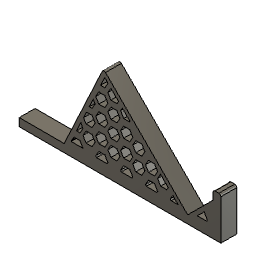
textbook holder fusion (Autodesk Fusion 360 design; units mm, degrees)
Autodesk Fusion 360 part; units mm, degrees
ref_plane "WorkPlane1" through (0, 0, 12.125) normal (0.707107, 0.707107, 0) x (0, 0, 1)
sketch "Sketch3" plane through (0, 0, 0) normal (0.707107, 0.707107, 0) x (0, 0, 1)
  line L0 (-200, 150) -> (200, 150)
  line L1 (200, 150) -> (200, -150)
  line L2 (200, -150) -> (-200, -150)
  line L3 (-200, -150) -> (-200, 150)
  line L4 (-200, 150) -> (200, -150) construction
  line L5 (200, 150) -> (-200, -150) construction
  point P0 (0, 116.066)
  point P1 (0, 116.066)
  dimension "d2" = 400
  dimension "d3" = 300
  constraint horizontal L0
  constraint perpendicular L0 L1
  constraint parallel L0 L2
  constraint parallel L1 L3
  constraint coincident L4 origin
  constraint coincident L5 origin
  measures "d2" distance of L1.end L2.end
  measures "d3" distance of L0.end L1.end
extrude "Extrude1" add sketch "Sketch3" along normal blind 45 makes body 1
sketch "Sketch4" plane through (0, 0, 0) normal (0, 1, 0) x (1, 0, 0)
  line L0 (106.066, 200) -> (106.066, -200)
move_body "Move1" bodies 1 to x (1, 0, 0) y (0, 1, 0) z (0, 0, 1) at (0, 106.066, 0)
move_body "Move2" bodies 1 to x (1, 0, 0) y (0, 1, 0) z (0, 0, 1) at (0, 10, 0)
sketch "Sketch5" plane through (0, 0, 0) normal (0, 1, 0) x (1, 0, 0)
  line L0 (106.066, -200) -> (-106.066, -200)
  line L1 (-106.066, 200) -> (106.066, 200)
  line L2 (106.066, -200) -> (137.8858, -200)
  line L3 (106.066, 200) -> (137.8858, 200)
  line L4 (-106.066, -200) -> (-106.066, 200)
  line L5 (137.8858, -200) -> (137.8858, 200)
  line L6 (-106.066, -180) -> (147.8858, -180)
  line L7 (147.8858, 180) -> (-106.066, 180)
  line L8 (137.8858, 200) -> (147.8858, 200)
  line L9 (137.8858, -200) -> (147.8858, -200)
  line L10 (147.8858, -200) -> (147.8858, 200)
  dimension "d9" = 20
  dimension "d10" = 20
  dimension "d13" = 10
  dimension "d14" = 10
  constraint coincident L4 L6.start
  constraint perpendicular L5 L6
  constraint coincident L4 L7.end
  constraint perpendicular L4 L7
  constraint coincident L3.end L5.end
  constraint perpendicular L5 L8
  constraint coincident L2.end L5.start
  constraint perpendicular L5 L9
  constraint coincident L10 L6.end
  constraint coincident L10 L7.start
  measures "d9" distance of L1 L7
  measures "d10" distance of L0 L6
  measures "d13" distance of L3.end L8.end
  measures "d14" distance of L2.end L9.end
extrude "Extrude2" add sketch "Sketch5" along normal blind 10 separate body contours L1 L3 L4 L5 L7 | L5 L7 L8 L10 makes body 2
sketch "Sketch6" plane through (0, 10, 0) normal (0, 1, 0) x (-1, 0, 0)
  line L0 (-147.8858, -180) -> (-147.8858, -200)
  line L1 (-147.8858, -200) -> (106.066, -200)
  line L2 (106.066, -200) -> (106.066, -180)
  line L3 (106.066, -180) -> (-147.8858, -180)
  line L4 (-147.8858, -180) -> (-137.8858, -180)
  line L5 (-137.8858, -180) -> (-137.8858, -200)
  line L6 (-137.8858, -200) -> (-147.8858, -200)
  line L7 (-147.8858, -200) -> (-147.8858, -180)
  dimension "d15" = 10
  constraint horizontal L4
  constraint vertical L5
  constraint horizontal L6
  constraint vertical L7
  constraint coincident L0.start L3.end
  measures "d15" distance of L0.start L4.end
extrude "Extrude3" add sketch "Sketch6" along normal blind 43.18 contours L0 L1 L3 L4 L5 L6 L7 bodies 2
sketch "Sketch7" plane through (0, 10, 0) normal (0, 1, 0) x (-1, 0, 0)
  line L0 (-137.8858, -180) -> (-137.8858, -200)
  line L1 (-137.8858, -200) -> (106.066, -200)
  line L2 (106.066, -180) -> (-137.8858, -180)
  line L3 (106.066, -180) -> (-137.8858, -180)
  line L4 (-137.8858, -200) -> (106.066, -200)
  line L5 (-133.1972, -180) -> (-133.1972, -200)
  line L6 (-123.4094, -200) -> (-123.4094, -180)
  line L7 (-123.4094, -184.92) -> (-133.1972, -184.92)
  line L8 (-133.1972, -190) -> (-123.4094, -190)
  line L9 (-123.4094, -195.08) -> (-133.1972, -195.08)
  line L10 (-133.1972, -180) -> (-123.4094, -180)
  line L11 (-128.3033, -180) -> (-128.3033, -200)
  line L12 (106.066, -200) -> (106.066, -180)
  point P0 (-128.3033, -184.92)
  point P1 (-128.3033, -190)
  point P2 (-128.3033, -195.08)
  dimension "d18" = 5.08
  dimension "d19" = 5.08
  constraint coincident L2.start L3.start
  constraint coincident L0.start L2.end
  constraint coincident L0.end L1.start
  constraint coincident L1.end L4.end
  constraint coincident L2 L5.start
  constraint coincident L4 L5.end
  constraint perpendicular L4 L5
  constraint coincident L1 L6.start
  constraint coincident L2 L6.end
  constraint perpendicular L2 L6
  constraint coincident L6 L7.start
  constraint coincident L5 L7.end
  constraint perpendicular L5 L7
  constraint midpoint L5 L8.start
  constraint midpoint L6 L8.end
  constraint coincident L6 L9.start
  constraint coincident L5 L9.end
  constraint perpendicular L5 L9
  constraint midpoint L10 L11.start
  constraint coincident L1 L11.end
  constraint perpendicular L1 L11
  constraint midpoint L7 P0
  constraint midpoint L8 P1
  constraint midpoint L9 P2
  measures "d18" distance of L7 L8
  measures "d19" distance of L8 L9
ref_plane "WorkPlane2" through (128.3033, 10, -190) normal (0, 0, -1) x (-1, 0, 0)
sketch "Sketch8" plane through (128.3033, 10, -190) normal (0, 0, -1) x (-1, 0, 0)
  line L0 (22.2373, 0) -> (-9.5825, 31.8198)
  line L1 (-9.5825, 0) -> (-9.5825, 43.18)
  line L2 (-9.5825, 0) -> (234.3693, 0)
  line L3 (234.3693, 212.132) -> (22.2373, 0)
  line L4 (-9.5825, 0) -> (234.3693, 0)
  line L5 (128.3033, 106.066) -> (22.2373, 0)
  line L6 (128.3033, 106.066) -> (177.7627, 0)
  dimension "d24" = 45
  dimension "d25" = 150
  dimension "d26" = 65
  constraint coincident L4 L0.start
  constraint coincident L0.start L3.end
  constraint coincident L2 L6.end
  measures "d24" angle of L4 L5
  measures "d25" distance of L5.start L0.start
  measures "d26" angle of L4 L6
extrude "Extrude5" add sketch "Sketch8" along normal mid plane 20 bodies 2
sketch "Sketch9" plane through (0, 0, -200) normal (0, 0, -1) x (-1, 0, 0)
  line L0 (49.4594, 10) -> (0, 116.066)
  line L1 (0, 116.066) -> (-106.066, 10)
  line L2 (53.2694, 3.4009) -> (57.0794, 10)
  line L3 (57.0794, 10) -> (53.2694, 16.5991)
  line L4 (53.2694, 16.5991) -> (45.6494, 16.5991)
  line L5 (45.6494, 16.5991) -> (41.8394, 10)
  line L6 (41.8394, 10) -> (45.6494, 3.4009)
  line L7 (45.6494, 3.4009) -> (53.2694, 3.4009)
  line L8 (41.611, 15) -> (-1.5137, 107.4812)
  line L9 (-1.5137, 107.4812) -> (-93.9949, 15)
  line L10 (-93.9949, 15) -> (41.611, 15)
  line L11 (-106.066, 10) -> (-137.8858, 41.8198)
  line L12 (-132.8858, 15) -> (-118.1371, 15)
  line L13 (-118.1371, 15) -> (-132.8858, 29.7487)
  line L14 (-132.8858, 29.7487) -> (-132.8858, 15)
  line L15 (29.6006, 10) -> (37.2206, 10)
  line L16 (37.2206, 10) -> (41.0306, 16.5991)
  line L17 (41.0306, 16.5991) -> (37.2206, 23.1982)
  line L18 (37.2206, 23.1982) -> (29.6006, 23.1982)
  line L19 (29.6006, 23.1982) -> (25.7906, 16.5991)
  line L20 (25.7906, 16.5991) -> (29.6006, 10)
  line L21 (106.066, 0) -> (-147.8858, 0)
  line L22 (45.6494, 16.5991) -> (23.7329, 16.5991)
  line L23 (14.3227, 16.5991) -> (10.5127, 10)
  line L24 (10.5127, 10) -> (14.3227, 3.4009)
  line L25 (14.3227, 3.4009) -> (21.9427, 3.4009)
  line L26 (21.9427, 3.4009) -> (25.7527, 10)
  line L27 (25.7527, 10) -> (21.9427, 16.5991)
  line L28 (21.9427, 16.5991) -> (14.3227, 16.5991)
  line L29 (-17.0039, 16.5991) -> (-20.8139, 10)
  line L30 (-20.8139, 10) -> (-17.0039, 3.4009)
  line L31 (-17.0039, 3.4009) -> (-9.3839, 3.4009)
  line L32 (-9.3839, 3.4009) -> (-5.5739, 10)
  line L33 (-5.5739, 10) -> (-9.3839, 16.5991)
  line L34 (-9.3839, 16.5991) -> (-17.0039, 16.5991)
  line L35 (-48.3306, 16.5991) -> (-52.1406, 10)
  line L36 (-52.1406, 10) -> (-48.3306, 3.4009)
  line L37 (-48.3306, 3.4009) -> (-40.7106, 3.4009)
  line L38 (-40.7106, 3.4009) -> (-36.9006, 10)
  line L39 (-36.9006, 10) -> (-40.7106, 16.5991)
  line L40 (-40.7106, 16.5991) -> (-48.3306, 16.5991)
  line L41 (-79.6573, 16.5991) -> (-83.4673, 10)
  line L42 (-83.4673, 10) -> (-79.6573, 3.4009)
  line L43 (-79.6573, 3.4009) -> (-72.0373, 3.4009)
  line L44 (-72.0373, 3.4009) -> (-68.2273, 10)
  line L45 (-68.2273, 10) -> (-72.0373, 16.5991)
  line L46 (-72.0373, 16.5991) -> (-79.6573, 16.5991)
  line L47 (-110.9839, 16.5991) -> (-114.7939, 10)
  line L48 (-114.7939, 10) -> (-110.9839, 3.4009)
  line L49 (-110.9839, 3.4009) -> (-103.3639, 3.4009)
  line L50 (-103.3639, 3.4009) -> (-99.5539, 10)
  line L51 (-99.5539, 10) -> (-103.3639, 16.5991)
  line L52 (-103.3639, 16.5991) -> (-110.9839, 16.5991)
  line L53 (-142.3106, 16.5991) -> (-146.1206, 10)
  line L54 (-146.1206, 10) -> (-142.3106, 3.4009)
  line L55 (-142.3106, 3.4009) -> (-134.6906, 3.4009)
  line L56 (-134.6906, 3.4009) -> (-130.8806, 10)
  line L57 (-130.8806, 10) -> (-134.6906, 16.5991)
  line L58 (-134.6906, 16.5991) -> (-142.3106, 16.5991)
  line L59 (45.6494, 37.4271) -> (41.8394, 30.828)
  line L60 (41.8394, 30.828) -> (45.6494, 24.2289)
  line L61 (45.6494, 24.2289) -> (53.2694, 24.2289)
  line L62 (53.2694, 24.2289) -> (57.0794, 30.828)
  line L63 (57.0794, 30.828) -> (53.2694, 37.4271)
  line L64 (53.2694, 37.4271) -> (45.6494, 37.4271)
  line L65 (14.3227, 37.4271) -> (10.5127, 30.828)
  line L66 (10.5127, 30.828) -> (14.3227, 24.2289)
  line L67 (14.3227, 24.2289) -> (21.9427, 24.2289)
  line L68 (21.9427, 24.2289) -> (25.7527, 30.828)
  line L69 (25.7527, 30.828) -> (21.9427, 37.4271)
  line L70 (21.9427, 37.4271) -> (14.3227, 37.4271)
  line L71 (-17.0039, 37.4271) -> (-20.8139, 30.828)
  line L72 (-20.8139, 30.828) -> (-17.0039, 24.2289)
  line L73 (-17.0039, 24.2289) -> (-9.3839, 24.2289)
  line L74 (-9.3839, 24.2289) -> (-5.5739, 30.828)
  line L75 (-5.5739, 30.828) -> (-9.3839, 37.4271)
  line L76 (-9.3839, 37.4271) -> (-17.0039, 37.4271)
  line L77 (-48.3306, 37.4271) -> (-52.1406, 30.828)
  line L78 (-52.1406, 30.828) -> (-48.3306, 24.2289)
  line L79 (-48.3306, 24.2289) -> (-40.7106, 24.2289)
  line L80 (-40.7106, 24.2289) -> (-36.9006, 30.828)
  line L81 (-36.9006, 30.828) -> (-40.7106, 37.4271)
  line L82 (-40.7106, 37.4271) -> (-48.3306, 37.4271)
  line L83 (-79.6573, 37.4271) -> (-83.4673, 30.828)
  line L84 (-83.4673, 30.828) -> (-79.6573, 24.2289)
  line L85 (-79.6573, 24.2289) -> (-72.0373, 24.2289)
  line L86 (-72.0373, 24.2289) -> (-68.2273, 30.828)
  line L87 (-68.2273, 30.828) -> (-72.0373, 37.4271)
  line L88 (-72.0373, 37.4271) -> (-79.6573, 37.4271)
  line L89 (-110.9839, 37.4271) -> (-114.7939, 30.828)
  line L90 (-114.7939, 30.828) -> (-110.9839, 24.2289)
  line L91 (-110.9839, 24.2289) -> (-103.3639, 24.2289)
  line L92 (-103.3639, 24.2289) -> (-99.5539, 30.828)
  line L93 (-99.5539, 30.828) -> (-103.3639, 37.4271)
  line L94 (-103.3639, 37.4271) -> (-110.9839, 37.4271)
  line L95 (-142.3106, 37.4271) -> (-146.1206, 30.828)
  line L96 (-146.1206, 30.828) -> (-142.3106, 24.2289)
  line L97 (-142.3106, 24.2289) -> (-134.6906, 24.2289)
  line L98 (-134.6906, 24.2289) -> (-130.8806, 30.828)
  line L99 (-130.8806, 30.828) -> (-134.6906, 37.4271)
  line L100 (-134.6906, 37.4271) -> (-142.3106, 37.4271)
  line L101 (45.6494, 58.2551) -> (41.8394, 51.656)
  line L102 (41.8394, 51.656) -> (45.6494, 45.0569)
  line L103 (45.6494, 45.0569) -> (53.2694, 45.0569)
  line L104 (53.2694, 45.0569) -> (57.0794, 51.656)
  line L105 (57.0794, 51.656) -> (53.2694, 58.2551)
  line L106 (53.2694, 58.2551) -> (45.6494, 58.2551)
  line L107 (14.3227, 58.2551) -> (10.5127, 51.656)
  line L108 (10.5127, 51.656) -> (14.3227, 45.0569)
  line L109 (14.3227, 45.0569) -> (21.9427, 45.0569)
  line L110 (21.9427, 45.0569) -> (25.7527, 51.656)
  line L111 (25.7527, 51.656) -> (21.9427, 58.2551)
  line L112 (21.9427, 58.2551) -> (14.3227, 58.2551)
  line L113 (-17.0039, 58.2551) -> (-20.8139, 51.656)
  line L114 (-20.8139, 51.656) -> (-17.0039, 45.0569)
  line L115 (-17.0039, 45.0569) -> (-9.3839, 45.0569)
  line L116 (-9.3839, 45.0569) -> (-5.5739, 51.656)
  line L117 (-5.5739, 51.656) -> (-9.3839, 58.2551)
  line L118 (-9.3839, 58.2551) -> (-17.0039, 58.2551)
  line L119 (-48.3306, 58.2551) -> (-52.1406, 51.656)
  line L120 (-52.1406, 51.656) -> (-48.3306, 45.0569)
  line L121 (-48.3306, 45.0569) -> (-40.7106, 45.0569)
  line L122 (-40.7106, 45.0569) -> (-36.9006, 51.656)
  line L123 (-36.9006, 51.656) -> (-40.7106, 58.2551)
  line L124 (-40.7106, 58.2551) -> (-48.3306, 58.2551)
  line L125 (-79.6573, 58.2551) -> (-83.4673, 51.656)
  line L126 (-83.4673, 51.656) -> (-79.6573, 45.0569)
  line L127 (-79.6573, 45.0569) -> (-72.0373, 45.0569)
  line L128 (-72.0373, 45.0569) -> (-68.2273, 51.656)
  line L129 (-68.2273, 51.656) -> (-72.0373, 58.2551)
  line L130 (-72.0373, 58.2551) -> (-79.6573, 58.2551)
  line L131 (-110.9839, 58.2551) -> (-114.7939, 51.656)
  line L132 (-114.7939, 51.656) -> (-110.9839, 45.0569)
  line L133 (-110.9839, 45.0569) -> (-103.3639, 45.0569)
  line L134 (-103.3639, 45.0569) -> (-99.5539, 51.656)
  line L135 (-99.5539, 51.656) -> (-103.3639, 58.2551)
  line L136 (-103.3639, 58.2551) -> (-110.9839, 58.2551)
  line L137 (-142.3106, 58.2551) -> (-146.1206, 51.656)
  line L138 (-146.1206, 51.656) -> (-142.3106, 45.0569)
  line L139 (-142.3106, 45.0569) -> (-134.6906, 45.0569)
  line L140 (-134.6906, 45.0569) -> (-130.8806, 51.656)
  line L141 (-130.8806, 51.656) -> (-134.6906, 58.2551)
  line L142 (-134.6906, 58.2551) -> (-142.3106, 58.2551)
  line L143 (45.6494, 79.0831) -> (41.8394, 72.484)
  line L144 (41.8394, 72.484) -> (45.6494, 65.8849)
  line L145 (45.6494, 65.8849) -> (53.2694, 65.8849)
  line L146 (53.2694, 65.8849) -> (57.0794, 72.484)
  line L147 (57.0794, 72.484) -> (53.2694, 79.0831)
  line L148 (53.2694, 79.0831) -> (45.6494, 79.0831)
  line L149 (14.3227, 79.0831) -> (10.5127, 72.484)
  line L150 (10.5127, 72.484) -> (14.3227, 65.8849)
  line L151 (14.3227, 65.8849) -> (21.9427, 65.8849)
  line L152 (21.9427, 65.8849) -> (25.7527, 72.484)
  line L153 (25.7527, 72.484) -> (21.9427, 79.0831)
  line L154 (21.9427, 79.0831) -> (14.3227, 79.0831)
  line L155 (-17.0039, 79.0831) -> (-20.8139, 72.484)
  line L156 (-20.8139, 72.484) -> (-17.0039, 65.8849)
  line L157 (-17.0039, 65.8849) -> (-9.3839, 65.8849)
  line L158 (-9.3839, 65.8849) -> (-5.5739, 72.484)
  line L159 (-5.5739, 72.484) -> (-9.3839, 79.0831)
  line L160 (-9.3839, 79.0831) -> (-17.0039, 79.0831)
  line L161 (-48.3306, 79.0831) -> (-52.1406, 72.484)
  line L162 (-52.1406, 72.484) -> (-48.3306, 65.8849)
  line L163 (-48.3306, 65.8849) -> (-40.7106, 65.8849)
  line L164 (-40.7106, 65.8849) -> (-36.9006, 72.484)
  line L165 (-36.9006, 72.484) -> (-40.7106, 79.0831)
  line L166 (-40.7106, 79.0831) -> (-48.3306, 79.0831)
  line L167 (-79.6573, 79.0831) -> (-83.4673, 72.484)
  line L168 (-83.4673, 72.484) -> (-79.6573, 65.8849)
  line L169 (-79.6573, 65.8849) -> (-72.0373, 65.8849)
  line L170 (-72.0373, 65.8849) -> (-68.2273, 72.484)
  line L171 (-68.2273, 72.484) -> (-72.0373, 79.0831)
  line L172 (-72.0373, 79.0831) -> (-79.6573, 79.0831)
  line L173 (-110.9839, 79.0831) -> (-114.7939, 72.484)
  line L174 (-114.7939, 72.484) -> (-110.9839, 65.8849)
  line L175 (-110.9839, 65.8849) -> (-103.3639, 65.8849)
  line L176 (-103.3639, 65.8849) -> (-99.5539, 72.484)
  line L177 (-99.5539, 72.484) -> (-103.3639, 79.0831)
  line L178 (-103.3639, 79.0831) -> (-110.9839, 79.0831)
  line L179 (-142.3106, 79.0831) -> (-146.1206, 72.484)
  line L180 (-146.1206, 72.484) -> (-142.3106, 65.8849)
  line L181 (-142.3106, 65.8849) -> (-134.6906, 65.8849)
  line L182 (-134.6906, 65.8849) -> (-130.8806, 72.484)
  line L183 (-130.8806, 72.484) -> (-134.6906, 79.0831)
  line L184 (-134.6906, 79.0831) -> (-142.3106, 79.0831)
  line L185 (45.6494, 99.9111) -> (41.8394, 93.312)
  line L186 (41.8394, 93.312) -> (45.6494, 86.7129)
  line L187 (45.6494, 86.7129) -> (53.2694, 86.7129)
  line L188 (53.2694, 86.7129) -> (57.0794, 93.312)
  line L189 (57.0794, 93.312) -> (53.2694, 99.9111)
  line L190 (53.2694, 99.9111) -> (45.6494, 99.9111)
  line L191 (14.3227, 99.9111) -> (10.5127, 93.312)
  line L192 (10.5127, 93.312) -> (14.3227, 86.7129)
  line L193 (14.3227, 86.7129) -> (21.9427, 86.7129)
  line L194 (21.9427, 86.7129) -> (25.7527, 93.312)
  line L195 (25.7527, 93.312) -> (21.9427, 99.9111)
  line L196 (21.9427, 99.9111) -> (14.3227, 99.9111)
  line L197 (-17.0039, 99.9111) -> (-20.8139, 93.312)
  line L198 (-20.8139, 93.312) -> (-17.0039, 86.7129)
  line L199 (-17.0039, 86.7129) -> (-9.3839, 86.7129)
  line L200 (-9.3839, 86.7129) -> (-5.5739, 93.312)
  line L201 (-5.5739, 93.312) -> (-9.3839, 99.9111)
  line L202 (-9.3839, 99.9111) -> (-17.0039, 99.9111)
  line L203 (-48.3306, 99.9111) -> (-52.1406, 93.312)
  line L204 (-52.1406, 93.312) -> (-48.3306, 86.7129)
  line L205 (-48.3306, 86.7129) -> (-40.7106, 86.7129)
  line L206 (-40.7106, 86.7129) -> (-36.9006, 93.312)
  line L207 (-36.9006, 93.312) -> (-40.7106, 99.9111)
  line L208 (-40.7106, 99.9111) -> (-48.3306, 99.9111)
  line L209 (-79.6573, 99.9111) -> (-83.4673, 93.312)
  line L210 (-83.4673, 93.312) -> (-79.6573, 86.7129)
  line L211 (-79.6573, 86.7129) -> (-72.0373, 86.7129)
  line L212 (-72.0373, 86.7129) -> (-68.2273, 93.312)
  line L213 (-68.2273, 93.312) -> (-72.0373, 99.9111)
  line L214 (-72.0373, 99.9111) -> (-79.6573, 99.9111)
  line L215 (-110.9839, 99.9111) -> (-114.7939, 93.312)
  line L216 (-114.7939, 93.312) -> (-110.9839, 86.7129)
  line L217 (-110.9839, 86.7129) -> (-103.3639, 86.7129)
  line L218 (-103.3639, 86.7129) -> (-99.5539, 93.312)
  line L219 (-99.5539, 93.312) -> (-103.3639, 99.9111)
  line L220 (-103.3639, 99.9111) -> (-110.9839, 99.9111)
  line L221 (-142.3106, 99.9111) -> (-146.1206, 93.312)
  line L222 (-146.1206, 93.312) -> (-142.3106, 86.7129)
  line L223 (-142.3106, 86.7129) -> (-134.6906, 86.7129)
  line L224 (-134.6906, 86.7129) -> (-130.8806, 93.312)
  line L225 (-130.8806, 93.312) -> (-134.6906, 99.9111)
  line L226 (-134.6906, 99.9111) -> (-142.3106, 99.9111)
  line L227 (45.6494, 120.7391) -> (41.8394, 114.14)
  line L228 (41.8394, 114.14) -> (45.6494, 107.5409)
  line L229 (45.6494, 107.5409) -> (53.2694, 107.5409)
  line L230 (53.2694, 107.5409) -> (57.0794, 114.14)
  line L231 (57.0794, 114.14) -> (53.2694, 120.7391)
  line L232 (53.2694, 120.7391) -> (45.6494, 120.7391)
  line L233 (14.3227, 120.7391) -> (10.5127, 114.14)
  line L234 (10.5127, 114.14) -> (14.3227, 107.5409)
  line L235 (14.3227, 107.5409) -> (21.9427, 107.5409)
  line L236 (21.9427, 107.5409) -> (25.7527, 114.14)
  line L237 (25.7527, 114.14) -> (21.9427, 120.7391)
  line L238 (21.9427, 120.7391) -> (14.3227, 120.7391)
  line L239 (-17.0039, 120.7391) -> (-20.8139, 114.14)
  line L240 (-20.8139, 114.14) -> (-17.0039, 107.5409)
  line L241 (-17.0039, 107.5409) -> (-9.3839, 107.5409)
  line L242 (-9.3839, 107.5409) -> (-5.5739, 114.14)
  line L243 (-5.5739, 114.14) -> (-9.3839, 120.7391)
  line L244 (-9.3839, 120.7391) -> (-17.0039, 120.7391)
  line L245 (-48.3306, 120.7391) -> (-52.1406, 114.14)
  line L246 (-52.1406, 114.14) -> (-48.3306, 107.5409)
  line L247 (-48.3306, 107.5409) -> (-40.7106, 107.5409)
  line L248 (-40.7106, 107.5409) -> (-36.9006, 114.14)
  line L249 (-36.9006, 114.14) -> (-40.7106, 120.7391)
  line L250 (-40.7106, 120.7391) -> (-48.3306, 120.7391)
  line L251 (-79.6573, 120.7391) -> (-83.4673, 114.14)
  line L252 (-83.4673, 114.14) -> (-79.6573, 107.5409)
  line L253 (-79.6573, 107.5409) -> (-72.0373, 107.5409)
  line L254 (-72.0373, 107.5409) -> (-68.2273, 114.14)
  line L255 (-68.2273, 114.14) -> (-72.0373, 120.7391)
  line L256 (-72.0373, 120.7391) -> (-79.6573, 120.7391)
  line L257 (-110.9839, 120.7391) -> (-114.7939, 114.14)
  line L258 (-114.7939, 114.14) -> (-110.9839, 107.5409)
  line L259 (-110.9839, 107.5409) -> (-103.3639, 107.5409)
  line L260 (-103.3639, 107.5409) -> (-99.5539, 114.14)
  line L261 (-99.5539, 114.14) -> (-103.3639, 120.7391)
  line L262 (-103.3639, 120.7391) -> (-110.9839, 120.7391)
  line L263 (-142.3106, 120.7391) -> (-146.1206, 114.14)
  line L264 (-146.1206, 114.14) -> (-142.3106, 107.5409)
  line L265 (-142.3106, 107.5409) -> (-134.6906, 107.5409)
  line L266 (-134.6906, 107.5409) -> (-130.8806, 114.14)
  line L267 (-130.8806, 114.14) -> (-134.6906, 120.7391)
  line L268 (-134.6906, 120.7391) -> (-142.3106, 120.7391)
  line L269 (-1.7261, 10) -> (5.8939, 10)
  line L270 (-5.5361, 16.5991) -> (-1.7261, 10)
  line L271 (5.8939, 23.1982) -> (-1.7261, 23.1982)
  line L272 (9.7039, 16.5991) -> (5.8939, 23.1982)
  line L273 (-1.7261, 23.1982) -> (-5.5361, 16.5991)
  line L274 (5.8939, 10) -> (9.7039, 16.5991)
  line L275 (-33.0527, 10) -> (-25.4327, 10)
  line L276 (-36.8627, 16.5991) -> (-33.0527, 10)
  line L277 (-25.4327, 23.1982) -> (-33.0527, 23.1982)
  line L278 (-21.6227, 16.5991) -> (-25.4327, 23.1982)
  line L279 (-33.0527, 23.1982) -> (-36.8627, 16.5991)
  line L280 (-25.4327, 10) -> (-21.6227, 16.5991)
  line L281 (-64.3794, 10) -> (-56.7594, 10)
  line L282 (-68.1894, 16.5991) -> (-64.3794, 10)
  line L283 (-56.7594, 23.1982) -> (-64.3794, 23.1982)
  line L284 (-52.9494, 16.5991) -> (-56.7594, 23.1982)
  line L285 (-64.3794, 23.1982) -> (-68.1894, 16.5991)
  line L286 (-56.7594, 10) -> (-52.9494, 16.5991)
  line L287 (-95.7061, 10) -> (-88.0861, 10)
  line L288 (-99.5161, 16.5991) -> (-95.7061, 10)
  line L289 (-88.0861, 23.1982) -> (-95.7061, 23.1982)
  line L290 (-84.2761, 16.5991) -> (-88.0861, 23.1982)
  line L291 (-95.7061, 23.1982) -> (-99.5161, 16.5991)
  line L292 (-88.0861, 10) -> (-84.2761, 16.5991)
  line L293 (-127.0327, 10) -> (-119.4127, 10)
  line L294 (-130.8427, 16.5991) -> (-127.0327, 10)
  line L295 (-119.4127, 23.1982) -> (-127.0327, 23.1982)
  line L296 (-115.6027, 16.5991) -> (-119.4127, 23.1982)
  line L297 (-127.0327, 23.1982) -> (-130.8427, 16.5991)
  line L298 (-119.4127, 10) -> (-115.6027, 16.5991)
  line L299 (-158.3594, 10) -> (-150.7394, 10)
  line L300 (-162.1694, 16.5991) -> (-158.3594, 10)
  line L301 (-150.7394, 23.1982) -> (-158.3594, 23.1982)
  line L302 (-146.9294, 16.5991) -> (-150.7394, 23.1982)
  line L303 (-158.3594, 23.1982) -> (-162.1694, 16.5991)
  line L304 (-150.7394, 10) -> (-146.9294, 16.5991)
  line L305 (29.6006, 31.59) -> (37.2206, 31.59)
  line L306 (25.7906, 38.1891) -> (29.6006, 31.59)
  line L307 (37.2206, 44.7882) -> (29.6006, 44.7882)
  line L308 (41.0306, 38.1891) -> (37.2206, 44.7882)
  line L309 (29.6006, 44.7882) -> (25.7906, 38.1891)
  line L310 (37.2206, 31.59) -> (41.0306, 38.1891)
  line L311 (-1.7261, 31.59) -> (5.8939, 31.59)
  line L312 (-5.5361, 38.1891) -> (-1.7261, 31.59)
  line L313 (5.8939, 44.7882) -> (-1.7261, 44.7882)
  line L314 (9.7039, 38.1891) -> (5.8939, 44.7882)
  line L315 (-1.7261, 44.7882) -> (-5.5361, 38.1891)
  line L316 (5.8939, 31.59) -> (9.7039, 38.1891)
  line L317 (-33.0527, 31.59) -> (-25.4327, 31.59)
  line L318 (-36.8627, 38.1891) -> (-33.0527, 31.59)
  line L319 (-25.4327, 44.7882) -> (-33.0527, 44.7882)
  line L320 (-21.6227, 38.1891) -> (-25.4327, 44.7882)
  line L321 (-33.0527, 44.7882) -> (-36.8627, 38.1891)
  line L322 (-25.4327, 31.59) -> (-21.6227, 38.1891)
  line L323 (-64.3794, 31.59) -> (-56.7594, 31.59)
  line L324 (-68.1894, 38.1891) -> (-64.3794, 31.59)
  line L325 (-56.7594, 44.7882) -> (-64.3794, 44.7882)
  line L326 (-52.9494, 38.1891) -> (-56.7594, 44.7882)
  line L327 (-64.3794, 44.7882) -> (-68.1894, 38.1891)
  line L328 (-56.7594, 31.59) -> (-52.9494, 38.1891)
  line L329 (-95.7061, 31.59) -> (-88.0861, 31.59)
  line L330 (-99.5161, 38.1891) -> (-95.7061, 31.59)
  line L331 (-88.0861, 44.7882) -> (-95.7061, 44.7882)
  line L332 (-84.2761, 38.1891) -> (-88.0861, 44.7882)
  line L333 (-95.7061, 44.7882) -> (-99.5161, 38.1891)
  line L334 (-88.0861, 31.59) -> (-84.2761, 38.1891)
  line L335 (-127.0327, 31.59) -> (-119.4127, 31.59)
  line L336 (-130.8427, 38.1891) -> (-127.0327, 31.59)
  line L337 (-119.4127, 44.7882) -> (-127.0327, 44.7882)
  line L338 (-115.6027, 38.1891) -> (-119.4127, 44.7882)
  line L339 (-127.0327, 44.7882) -> (-130.8427, 38.1891)
  line L340 (-119.4127, 31.59) -> (-115.6027, 38.1891)
  line L341 (-158.3594, 31.59) -> (-150.7394, 31.59)
  line L342 (-162.1694, 38.1891) -> (-158.3594, 31.59)
  line L343 (-150.7394, 44.7882) -> (-158.3594, 44.7882)
  line L344 (-146.9294, 38.1891) -> (-150.7394, 44.7882)
  line L345 (-158.3594, 44.7882) -> (-162.1694, 38.1891)
  line L346 (-150.7394, 31.59) -> (-146.9294, 38.1891)
  line L347 (29.6006, 53.18) -> (37.2206, 53.18)
  line L348 (25.7906, 59.7791) -> (29.6006, 53.18)
  line L349 (37.2206, 66.3782) -> (29.6006, 66.3782)
  line L350 (41.0306, 59.7791) -> (37.2206, 66.3782)
  line L351 (29.6006, 66.3782) -> (25.7906, 59.7791)
  line L352 (37.2206, 53.18) -> (41.0306, 59.7791)
  line L353 (-1.7261, 53.18) -> (5.8939, 53.18)
  line L354 (-5.5361, 59.7791) -> (-1.7261, 53.18)
  line L355 (5.8939, 66.3782) -> (-1.7261, 66.3782)
  line L356 (9.7039, 59.7791) -> (5.8939, 66.3782)
  line L357 (-1.7261, 66.3782) -> (-5.5361, 59.7791)
  line L358 (5.8939, 53.18) -> (9.7039, 59.7791)
  line L359 (-33.0527, 53.18) -> (-25.4327, 53.18)
  line L360 (-36.8627, 59.7791) -> (-33.0527, 53.18)
  line L361 (-25.4327, 66.3782) -> (-33.0527, 66.3782)
  line L362 (-21.6227, 59.7791) -> (-25.4327, 66.3782)
  line L363 (-33.0527, 66.3782) -> (-36.8627, 59.7791)
  line L364 (-25.4327, 53.18) -> (-21.6227, 59.7791)
  line L365 (-64.3794, 53.18) -> (-56.7594, 53.18)
  line L366 (-68.1894, 59.7791) -> (-64.3794, 53.18)
  line L367 (-56.7594, 66.3782) -> (-64.3794, 66.3782)
  line L368 (-52.9494, 59.7791) -> (-56.7594, 66.3782)
  line L369 (-64.3794, 66.3782) -> (-68.1894, 59.7791)
  line L370 (-56.7594, 53.18) -> (-52.9494, 59.7791)
  line L371 (-95.7061, 53.18) -> (-88.0861, 53.18)
  line L372 (-99.5161, 59.7791) -> (-95.7061, 53.18)
  line L373 (-88.0861, 66.3782) -> (-95.7061, 66.3782)
  line L374 (-84.2761, 59.7791) -> (-88.0861, 66.3782)
  line L375 (-95.7061, 66.3782) -> (-99.5161, 59.7791)
  line L376 (-88.0861, 53.18) -> (-84.2761, 59.7791)
  line L377 (-127.0327, 53.18) -> (-119.4127, 53.18)
  line L378 (-130.8427, 59.7791) -> (-127.0327, 53.18)
  line L379 (-119.4127, 66.3782) -> (-127.0327, 66.3782)
  line L380 (-115.6027, 59.7791) -> (-119.4127, 66.3782)
  line L381 (-127.0327, 66.3782) -> (-130.8427, 59.7791)
  line L382 (-119.4127, 53.18) -> (-115.6027, 59.7791)
  line L383 (-158.3594, 53.18) -> (-150.7394, 53.18)
  line L384 (-162.1694, 59.7791) -> (-158.3594, 53.18)
  line L385 (-150.7394, 66.3782) -> (-158.3594, 66.3782)
  line L386 (-146.9294, 59.7791) -> (-150.7394, 66.3782)
  line L387 (-158.3594, 66.3782) -> (-162.1694, 59.7791)
  line L388 (-150.7394, 53.18) -> (-146.9294, 59.7791)
  line L389 (29.6006, 74.77) -> (37.2206, 74.77)
  line L390 (25.7906, 81.3691) -> (29.6006, 74.77)
  line L391 (37.2206, 87.9682) -> (29.6006, 87.9682)
  line L392 (41.0306, 81.3691) -> (37.2206, 87.9682)
  line L393 (29.6006, 87.9682) -> (25.7906, 81.3691)
  line L394 (37.2206, 74.77) -> (41.0306, 81.3691)
  line L395 (-1.7261, 74.77) -> (5.8939, 74.77)
  line L396 (-5.5361, 81.3691) -> (-1.7261, 74.77)
  line L397 (5.8939, 87.9682) -> (-1.7261, 87.9682)
  line L398 (9.7039, 81.3691) -> (5.8939, 87.9682)
  line L399 (-1.7261, 87.9682) -> (-5.5361, 81.3691)
  line L400 (5.8939, 74.77) -> (9.7039, 81.3691)
  line L401 (-33.0527, 74.77) -> (-25.4327, 74.77)
  line L402 (-36.8627, 81.3691) -> (-33.0527, 74.77)
  line L403 (-25.4327, 87.9682) -> (-33.0527, 87.9682)
  line L404 (-21.6227, 81.3691) -> (-25.4327, 87.9682)
  line L405 (-33.0527, 87.9682) -> (-36.8627, 81.3691)
  line L406 (-25.4327, 74.77) -> (-21.6227, 81.3691)
  line L407 (-64.3794, 74.77) -> (-56.7594, 74.77)
  line L408 (-68.1894, 81.3691) -> (-64.3794, 74.77)
  line L409 (-56.7594, 87.9682) -> (-64.3794, 87.9682)
  line L410 (-52.9494, 81.3691) -> (-56.7594, 87.9682)
  line L411 (-64.3794, 87.9682) -> (-68.1894, 81.3691)
  line L412 (-56.7594, 74.77) -> (-52.9494, 81.3691)
  line L413 (-95.7061, 74.77) -> (-88.0861, 74.77)
  line L414 (-99.5161, 81.3691) -> (-95.7061, 74.77)
  line L415 (-88.0861, 87.9682) -> (-95.7061, 87.9682)
  line L416 (-84.2761, 81.3691) -> (-88.0861, 87.9682)
  line L417 (-95.7061, 87.9682) -> (-99.5161, 81.3691)
  line L418 (-88.0861, 74.77) -> (-84.2761, 81.3691)
  line L419 (-127.0327, 74.77) -> (-119.4127, 74.77)
  line L420 (-130.8427, 81.3691) -> (-127.0327, 74.77)
  line L421 (-119.4127, 87.9682) -> (-127.0327, 87.9682)
  line L422 (-115.6027, 81.3691) -> (-119.4127, 87.9682)
  line L423 (-127.0327, 87.9682) -> (-130.8427, 81.3691)
  line L424 (-119.4127, 74.77) -> (-115.6027, 81.3691)
  line L425 (-158.3594, 74.77) -> (-150.7394, 74.77)
  line L426 (-162.1694, 81.3691) -> (-158.3594, 74.77)
  line L427 (-150.7394, 87.9682) -> (-158.3594, 87.9682)
  line L428 (-146.9294, 81.3691) -> (-150.7394, 87.9682)
  line L429 (-158.3594, 87.9682) -> (-162.1694, 81.3691)
  line L430 (-150.7394, 74.77) -> (-146.9294, 81.3691)
  line L431 (29.6006, 96.36) -> (37.2206, 96.36)
  line L432 (25.7906, 102.9591) -> (29.6006, 96.36)
  line L433 (37.2206, 109.5582) -> (29.6006, 109.5582)
  line L434 (41.0306, 102.9591) -> (37.2206, 109.5582)
  line L435 (29.6006, 109.5582) -> (25.7906, 102.9591)
  line L436 (37.2206, 96.36) -> (41.0306, 102.9591)
  line L437 (-1.7261, 96.36) -> (5.8939, 96.36)
  line L438 (-5.5361, 102.9591) -> (-1.7261, 96.36)
  line L439 (5.8939, 109.5582) -> (-1.7261, 109.5582)
  line L440 (9.7039, 102.9591) -> (5.8939, 109.5582)
  line L441 (-1.7261, 109.5582) -> (-5.5361, 102.9591)
  line L442 (5.8939, 96.36) -> (9.7039, 102.9591)
  line L443 (-33.0527, 96.36) -> (-25.4327, 96.36)
  line L444 (-36.8627, 102.9591) -> (-33.0527, 96.36)
  line L445 (-25.4327, 109.5582) -> (-33.0527, 109.5582)
  line L446 (-21.6227, 102.9591) -> (-25.4327, 109.5582)
  line L447 (-33.0527, 109.5582) -> (-36.8627, 102.9591)
  line L448 (-25.4327, 96.36) -> (-21.6227, 102.9591)
  line L449 (-64.3794, 96.36) -> (-56.7594, 96.36)
  line L450 (-68.1894, 102.9591) -> (-64.3794, 96.36)
  line L451 (-56.7594, 109.5582) -> (-64.3794, 109.5582)
  line L452 (-52.9494, 102.9591) -> (-56.7594, 109.5582)
  line L453 (-64.3794, 109.5582) -> (-68.1894, 102.9591)
  line L454 (-56.7594, 96.36) -> (-52.9494, 102.9591)
  line L455 (-95.7061, 96.36) -> (-88.0861, 96.36)
  line L456 (-99.5161, 102.9591) -> (-95.7061, 96.36)
  line L457 (-88.0861, 109.5582) -> (-95.7061, 109.5582)
  line L458 (-84.2761, 102.9591) -> (-88.0861, 109.5582)
  line L459 (-95.7061, 109.5582) -> (-99.5161, 102.9591)
  line L460 (-88.0861, 96.36) -> (-84.2761, 102.9591)
  line L461 (-127.0327, 96.36) -> (-119.4127, 96.36)
  line L462 (-130.8427, 102.9591) -> (-127.0327, 96.36)
  line L463 (-119.4127, 109.5582) -> (-127.0327, 109.5582)
  line L464 (-115.6027, 102.9591) -> (-119.4127, 109.5582)
  line L465 (-127.0327, 109.5582) -> (-130.8427, 102.9591)
  line L466 (-119.4127, 96.36) -> (-115.6027, 102.9591)
  line L467 (-158.3594, 96.36) -> (-150.7394, 96.36)
  line L468 (-162.1694, 102.9591) -> (-158.3594, 96.36)
  line L469 (-150.7394, 109.5582) -> (-158.3594, 109.5582)
  line L470 (-146.9294, 102.9591) -> (-150.7394, 109.5582)
  line L471 (-158.3594, 109.5582) -> (-162.1694, 102.9591)
  line L472 (-150.7394, 96.36) -> (-146.9294, 102.9591)
  line L473 (29.6006, 117.95) -> (37.2206, 117.95)
  line L474 (25.7906, 124.5491) -> (29.6006, 117.95)
  line L475 (37.2206, 131.1482) -> (29.6006, 131.1482)
  line L476 (41.0306, 124.5491) -> (37.2206, 131.1482)
  line L477 (29.6006, 131.1482) -> (25.7906, 124.5491)
  line L478 (37.2206, 117.95) -> (41.0306, 124.5491)
  line L479 (-1.7261, 117.95) -> (5.8939, 117.95)
  line L480 (-5.5361, 124.5491) -> (-1.7261, 117.95)
  line L481 (5.8939, 131.1482) -> (-1.7261, 131.1482)
  line L482 (9.7039, 124.5491) -> (5.8939, 131.1482)
  line L483 (-1.7261, 131.1482) -> (-5.5361, 124.5491)
  line L484 (5.8939, 117.95) -> (9.7039, 124.5491)
  line L485 (-33.0527, 117.95) -> (-25.4327, 117.95)
  line L486 (-36.8627, 124.5491) -> (-33.0527, 117.95)
  line L487 (-25.4327, 131.1482) -> (-33.0527, 131.1482)
  line L488 (-21.6227, 124.5491) -> (-25.4327, 131.1482)
  line L489 (-33.0527, 131.1482) -> (-36.8627, 124.5491)
  line L490 (-25.4327, 117.95) -> (-21.6227, 124.5491)
  line L491 (-64.3794, 117.95) -> (-56.7594, 117.95)
  line L492 (-68.1894, 124.5491) -> (-64.3794, 117.95)
  line L493 (-56.7594, 131.1482) -> (-64.3794, 131.1482)
  line L494 (-52.9494, 124.5491) -> (-56.7594, 131.1482)
  line L495 (-64.3794, 131.1482) -> (-68.1894, 124.5491)
  line L496 (-56.7594, 117.95) -> (-52.9494, 124.5491)
  line L497 (-95.7061, 117.95) -> (-88.0861, 117.95)
  line L498 (-99.5161, 124.5491) -> (-95.7061, 117.95)
  line L499 (-88.0861, 131.1482) -> (-95.7061, 131.1482)
  line L500 (-84.2761, 124.5491) -> (-88.0861, 131.1482)
  line L501 (-95.7061, 131.1482) -> (-99.5161, 124.5491)
  line L502 (-88.0861, 117.95) -> (-84.2761, 124.5491)
  line L503 (-127.0327, 117.95) -> (-119.4127, 117.95)
  line L504 (-130.8427, 124.5491) -> (-127.0327, 117.95)
  line L505 (-119.4127, 131.1482) -> (-127.0327, 131.1482)
  line L506 (-115.6027, 124.5491) -> (-119.4127, 131.1482)
  line L507 (-127.0327, 131.1482) -> (-130.8427, 124.5491)
  line L508 (-119.4127, 117.95) -> (-115.6027, 124.5491)
  line L509 (-158.3594, 117.95) -> (-150.7394, 117.95)
  line L510 (-162.1694, 124.5491) -> (-158.3594, 117.95)
  line L511 (-150.7394, 131.1482) -> (-158.3594, 131.1482)
  line L512 (-146.9294, 124.5491) -> (-150.7394, 131.1482)
  line L513 (-158.3594, 131.1482) -> (-162.1694, 124.5491)
  line L514 (-150.7394, 117.95) -> (-146.9294, 124.5491)
  line L515 (29.6006, 139.54) -> (37.2206, 139.54)
  line L516 (25.7906, 146.1391) -> (29.6006, 139.54)
  line L517 (37.2206, 152.7382) -> (29.6006, 152.7382)
  line L518 (41.0306, 146.1391) -> (37.2206, 152.7382)
  line L519 (29.6006, 152.7382) -> (25.7906, 146.1391)
  line L520 (37.2206, 139.54) -> (41.0306, 146.1391)
  line L521 (-1.7261, 139.54) -> (5.8939, 139.54)
  line L522 (-5.5361, 146.1391) -> (-1.7261, 139.54)
  line L523 (5.8939, 152.7382) -> (-1.7261, 152.7382)
  line L524 (9.7039, 146.1391) -> (5.8939, 152.7382)
  line L525 (-1.7261, 152.7382) -> (-5.5361, 146.1391)
  line L526 (5.8939, 139.54) -> (9.7039, 146.1391)
  line L527 (-33.0527, 139.54) -> (-25.4327, 139.54)
  line L528 (-36.8627, 146.1391) -> (-33.0527, 139.54)
  line L529 (-25.4327, 152.7382) -> (-33.0527, 152.7382)
  line L530 (-21.6227, 146.1391) -> (-25.4327, 152.7382)
  line L531 (-33.0527, 152.7382) -> (-36.8627, 146.1391)
  line L532 (-25.4327, 139.54) -> (-21.6227, 146.1391)
  line L533 (-64.3794, 139.54) -> (-56.7594, 139.54)
  line L534 (-68.1894, 146.1391) -> (-64.3794, 139.54)
  line L535 (-56.7594, 152.7382) -> (-64.3794, 152.7382)
  line L536 (-52.9494, 146.1391) -> (-56.7594, 152.7382)
  line L537 (-64.3794, 152.7382) -> (-68.1894, 146.1391)
  line L538 (-56.7594, 139.54) -> (-52.9494, 146.1391)
  line L539 (-95.7061, 139.54) -> (-88.0861, 139.54)
  line L540 (-99.5161, 146.1391) -> (-95.7061, 139.54)
  line L541 (-88.0861, 152.7382) -> (-95.7061, 152.7382)
  line L542 (-84.2761, 146.1391) -> (-88.0861, 152.7382)
  line L543 (-95.7061, 152.7382) -> (-99.5161, 146.1391)
  line L544 (-88.0861, 139.54) -> (-84.2761, 146.1391)
  line L545 (-127.0327, 139.54) -> (-119.4127, 139.54)
  line L546 (-130.8427, 146.1391) -> (-127.0327, 139.54)
  line L547 (-119.4127, 152.7382) -> (-127.0327, 152.7382)
  line L548 (-115.6027, 146.1391) -> (-119.4127, 152.7382)
  line L549 (-127.0327, 152.7382) -> (-130.8427, 146.1391)
  line L550 (-119.4127, 139.54) -> (-115.6027, 146.1391)
  line L551 (-158.3594, 139.54) -> (-150.7394, 139.54)
  line L552 (-162.1694, 146.1391) -> (-158.3594, 139.54)
  line L553 (-150.7394, 152.7382) -> (-158.3594, 152.7382)
  line L554 (-146.9294, 146.1391) -> (-150.7394, 152.7382)
  line L555 (-158.3594, 152.7382) -> (-162.1694, 146.1391)
  line L556 (-150.7394, 139.54) -> (-146.9294, 146.1391)
  line L557 (-147.8858, 0) -> (106.066, 0)
  line L558 (106.066, 0) -> (106.066, 10)
  line L559 (106.066, 10) -> (49.4594, 10)
  line L560 (-106.066, 10) -> (-137.8858, 41.8198)
  line L561 (-137.8858, 41.8198) -> (-137.8858, 53.18)
  line L562 (-137.8858, 53.18) -> (-147.8858, 53.18)
  line L563 (-147.8858, 53.18) -> (-147.8858, 0)
  line L564 (-147.8858, 0) -> (106.066, 0)
  line L565 (106.066, 0) -> (106.066, 10)
  line L566 (106.066, 10) -> (49.4594, 10)
  line L567 (49.4594, 10) -> (0, 116.066)
  line L568 (0, 116.066) -> (-106.066, 10)
  line L569 (-137.8858, 41.8198) -> (-137.8858, 53.18)
  line L570 (-137.8858, 53.18) -> (-147.8858, 53.18)
  line L571 (-147.8858, 53.18) -> (-147.8858, 0)
  point P0 (49.4594, 10)
  point P1 (33.4106, 16.5991)
  point P2 (33.4106, 16.5991)
  point P3 (18.1327, 10)
  point P4 (-13.1939, 10)
  point P5 (-44.5206, 10)
  point P6 (-75.8473, 10)
  point P7 (-107.1739, 10)
  point P8 (-138.5006, 10)
  point P9 (49.4594, 30.828)
  point P10 (18.1327, 30.828)
  point P11 (-13.1939, 30.828)
  point P12 (-44.5206, 30.828)
  point P13 (-75.8473, 30.828)
  point P14 (-107.1739, 30.828)
  point P15 (-138.5006, 30.828)
  point P16 (49.4594, 51.656)
  point P17 (18.1327, 51.656)
  point P18 (-13.1939, 51.656)
  point P19 (-44.5206, 51.656)
  point P20 (-75.8473, 51.656)
  point P21 (-107.1739, 51.656)
  point P22 (-138.5006, 51.656)
  point P23 (49.4594, 72.484)
  point P24 (18.1327, 72.484)
  point P25 (-13.1939, 72.484)
  point P26 (-44.5206, 72.484)
  point P27 (-75.8473, 72.484)
  point P28 (-107.1739, 72.484)
  point P29 (-138.5006, 72.484)
  point P30 (49.4594, 93.312)
  point P31 (18.1327, 93.312)
  point P32 (-13.1939, 93.312)
  point P33 (-44.5206, 93.312)
  point P34 (-75.8473, 93.312)
  point P35 (-107.1739, 93.312)
  point P36 (-138.5006, 93.312)
  point P37 (49.4594, 114.14)
  point P38 (18.1327, 114.14)
  point P39 (-13.1939, 114.14)
  point P40 (-44.5206, 114.14)
  point P41 (-75.8473, 114.14)
  point P42 (-107.1739, 114.14)
  point P43 (-138.5006, 114.14)
  point P44 (2.0839, 16.5991)
  point P45 (-29.2427, 16.5991)
  point P46 (-60.5694, 16.5991)
  point P47 (-91.8961, 16.5991)
  point P48 (-123.2227, 16.5991)
  point P49 (-154.5494, 16.5991)
  point P50 (33.4106, 38.1891)
  point P51 (2.0839, 38.1891)
  point P52 (-29.2427, 38.1891)
  point P53 (-60.5694, 38.1891)
  point P54 (-91.8961, 38.1891)
  point P55 (-123.2227, 38.1891)
  point P56 (-154.5494, 38.1891)
  point P57 (33.4106, 59.7791)
  point P58 (2.0839, 59.7791)
  point P59 (-29.2427, 59.7791)
  point P60 (-60.5694, 59.7791)
  point P61 (-91.8961, 59.7791)
  point P62 (-123.2227, 59.7791)
  point P63 (-154.5494, 59.7791)
  point P64 (33.4106, 81.3691)
  point P65 (2.0839, 81.3691)
  point P66 (-29.2427, 81.3691)
  point P67 (-60.5694, 81.3691)
  point P68 (-91.8961, 81.3691)
  point P69 (-123.2227, 81.3691)
  point P70 (-154.5494, 81.3691)
  point P71 (33.4106, 102.9591)
  point P72 (2.0839, 102.9591)
  point P73 (-29.2427, 102.9591)
  point P74 (-60.5694, 102.9591)
  point P75 (-91.8961, 102.9591)
  point P76 (-123.2227, 102.9591)
  point P77 (-154.5494, 102.9591)
  point P78 (33.4106, 124.5491)
  point P79 (2.0839, 124.5491)
  point P80 (-29.2427, 124.5491)
  point P81 (-60.5694, 124.5491)
  point P82 (-91.8961, 124.5491)
  point P83 (-123.2227, 124.5491)
  point P84 (-154.5494, 124.5491)
  point P85 (33.4106, 146.1391)
  point P86 (2.0839, 146.1391)
  point P87 (-29.2427, 146.1391)
  point P88 (-60.5694, 146.1391)
  point P89 (-91.8961, 146.1391)
  point P90 (-123.2227, 146.1391)
  point P91 (-154.5494, 146.1391)
  dimension "d29" = 7.62
  dimension "d32" = 7.62
  dimension "d33" = 4
  dimension "d36" = -187.96
  dimension "d37" = 104.14
  dimension "d40" = -187.96
  dimension "d41" = 129.54
  constraint coincident P0 L0.start
  constraint parallel L15 L21
  constraint coincident P2 P1
  constraint parallel L4 L22
  constraint coincident P2 L22
  measures "d29" distance of L2.start L6.end
  measures "d32" distance of L15.start L15.end
  measures "d33" distance of L5 L16
extrude "Extrude6" cut sketch "Sketch9" against normal blind 68.58 contours L8 L305 L306 L309 | L8 L17 L18 L19 L22 | L8 L107 L108 L109 L110 L112 | L8 L149 L150 L151 | L10 L270 L271 L272 L273 L274 | L8 L9 L437 L438 L441 | L9 L198 L199 L200 L201 | L10 L276 L277 L278 L279 L280 | L9 L401 L402 L404 L406 | L10 L282 L283 L284 L285 L286 | L9 L323 L324 L325 L326 L327 L328 | L9 L10 L290 L292 | L9 L84 L85 L86 L87 | L12 L13 L294 L295 L297 | L65 L66 L67 L68 L69 L70 | L71 L72 L73 L74 L75 L76 | L77 L78 L79 L80 L81 L82 | L113 L114 L115 L116 L117 L118 | L119 L120 L121 L122 L123 L124 | L155 L156 L157 L158 L159 L160 | L311 L312 L313 L314 L315 L316 | L317 L318 L319 L320 L321 L322 | L353 L354 L355 L356 L357 L358 | L359 L360 L361 L362 L363 L364 | L395 L396 L397 L398 L399 L400 bodies 2
fillet "Fillet1" radius 2.54 3 edges at (147.8858, 53.18, -190) (137.8858, 53.18, -190) (0, 116.066, -190) on bodies 2
copy_body "CopyPasteBodies1" bodies 2 makes body 3
move_body "Move3" bodies 3 to x (1, 0, 0) y (0, 1, 0) z (0, 0, 1) at (0, 0, 381)
hidden bodies 1 3
equation "d2 = 200 * 2 mm"
named bodies: "book", "stand", "stand (1)"
